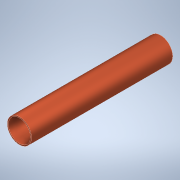
# Autodesk Inventor part: 4000_Cu_Bias_Shielding_(McMaster_50475K18)_MPSv2_v2
Saved by Autodesk Inventor 2021 (Build 250183000, 183)
## iProperties
Created: 2020-11-11
Part Number: 4000_Cu_Bias_Shielding_(McMaster_50475K18)_MPSv2_v2
Material: Copper
Document SubType Name: Modeling
Designer: Admin
Density: 8.94 g/cm^3
Appearance: Copper - Satin
Author: Admin
Autodesk Inventor part; units mm, degrees
ref_plane "YZ Plane" through (0, 0, 0) normal (1, 0, 0) x (0, 1, 0)
ref_plane "XZ Plane" through (0, 0, 0) normal (0, 1, 0) x (-1, 0, 0)
ref_plane "XY Plane" through (0, 0, 0) normal (0, 0, 1) x (1, 0, 0)
sketch "Sketch1" plane through (0, 0, 0) normal (0, 0, 1) x (1, 0, 0)
  circle A0 centre (0, 0) radius 18.8087
  circle A1 centre (0, 0) radius 20.6375
  dimension "d0" = 37.6174
  dimension "d1" = 41.275
  constraints: 2 centre point, 2 coincident
  measures "d0" diameter of A0
  measures "d1" diameter of A1
extrude "Extrusion1" add sketch "Sketch1" along normal blind 240
ref_plane "Work Plane1" through (-18.8087, 0, 0) normal (0, -1, 0) x (1, 0, 0)
body "Solid1"
